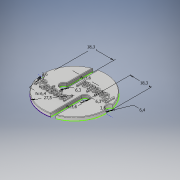
# Autodesk Inventor part: cookie_copied
Saved by Autodesk Inventor 2019 (Build 230136000, 136)
## iProperties
Created: 2019-04-04
Part Number: cookie_copied
Material: Generic
Document SubType Name: Modeling
Designer: jmc
Density: 1 g/cm^3
Appearance: Default
Author: jmc
## iProperties of the stored document cookie_copied_3DPrint.ipt
Created: 2019-04-04
Part Number: cookie_copied_3DPrint
Material: Generic
Document SubType Name: Modeling
Designer: assman
Density: 1 g/cm^3
Appearance: Default
Author: assman
Autodesk Inventor part; units mm, degrees
ref_plane "YZ Plane" through (0, 0, 0) normal (1, 0, 0) x (0, 1, 0)
ref_plane "XZ Plane" through (0, 0, 0) normal (0, 1, 0) x (-1, 0, 0)
ref_plane "XY Plane" through (0, 0, 0) normal (0, 0, 1) x (1, 0, 0)
sketch "Sketch1" plane through (0, 0, 0) normal (0, 1, 0) x (-1, 0, 0)
  line L0 (32.3118, 0) -> (-33.3424, 0) construction
  arc A0 (9.65, -3.1177) -> (6.05, 0) centre (9.2, 0) ccw
  arc A1 (-9.647, 3.1177) -> (-6.047, 0) centre (-9.197, 0) ccw
  line L1 (27.5, 0) -> (27.5, -9.7231) construction
  line L2 (-6.047, 0) -> (-6.047, 26.8269)
  line L3 (-9.647, 3.1177) -> (-9.647, 25.7524)
  arc A2 (-26.6628, -6.734) -> (-27.497, -0.4055) centre (-27.3093, -3.6) ccw
  arc A3 (26.6628, 6.7338) -> (27.497, 0.4054) centre (27.3103, 3.6) ccw
  arc A4 (-9.647, 25.7524) -> (-27.497, -0.4055) centre (0, 0) ccw
  arc A5 (-26.6628, -6.734) -> (6.05, -26.8262) centre (0, 0) ccw
  arc A6 (9.65, -25.7513) -> (27.497, 0.4054) centre (0, 0) ccw
  arc A7 (26.6628, 6.7338) -> (-6.047, 26.8269) centre (0, 0) ccw
  line L4 (-27.497, -0.4055) -> (-27.497, 9.5971) construction
  line L5 (6.05, 0) -> (6.05, -26.8262)
  line L6 (9.65, -25.7513) -> (9.65, -3.1177)
  point P0 (12.35, 0)
  dimension "d1" = 6.3
  dimension "d2" = 6.3
  dimension "d3" = 18.3
  dimension "d6" = 3.6
  dimension "d7" = 6.4
  dimension "d8" = 6.4
  dimension "d11" = 27.5
  dimension "d12" = 18.3
  dimension "d13" = 3.6
  dimension "d14" = 3.6
  dimension "d15" = 3.6
  constraints: 18 point on circle, 14 end point, 8 centre point, 6 point on line, 3 tangent, 3 vertical, 2 perpendicular, 1 coincident, 1 horizontal
  measures "d1" diameter of A0
  measures "d2" diameter of A1
  measures "d3" distance from line of L1 A0.centre
  measures "d6" distance between parallel lines of L2 L3
  measures "d7" diameter of A2
  measures "d8" diameter of A3
  measures "d11" radius of A7
  measures "d12" distance from line of L4 A1.centre
  measures "d13" distance from line of L0 A2.centre
  measures "d14" distance from line of A3.centre L0
  measures "d15" distance between parallel lines of L6 L5
extrude "Extrusion1" add sketch "Sketch1" along normal blind 2.8
sketch "Sketch2" plane through (0, 2.8, 0) normal (0, 1, 0) x (1, 0, 0)
  line L0 (-23.6967, -4.3993) -> (3.8634, -4.3993) construction
  line L1 (3.8634, -4.3993) -> (3.8634, -12.2502) construction
  line L2 (3.8634, -12.2502) -> (-23.6967, -12.2502) construction
  line L3 (-23.6967, -12.2502) -> (-23.6967, -4.3993) construction
  line L4 (23.6967, 4.719) -> (-3.8634, 4.719) construction
  line L5 (-3.8634, 4.719) -> (-3.8634, 12.5699) construction
  line L6 (-3.8634, 12.5699) -> (23.6967, 12.5699) construction
  line L7 (23.6967, 12.5699) -> (23.6967, 4.719) construction
  spline S0 degree 2 poles (-23.1038, -11.4801) (-23.1038, -11.6982) (-22.8993, -12.0662) (-22.654, -12.0798) knots 0 0 0 1 2 2 2
  spline S1 degree 2 poles (-22.654, -12.0798) (-22.3609, -12.0866) (-21.8771, -11.8617) (-21.8634, -11.5483) knots 0 0 0 1 2 2 2
  spline S2 degree 2 poles (-21.8634, -11.5483) (-21.8702, -11.4324) (-21.952, -11.2279) (-21.9793, -11.1666) knots 0 0 0 1 2 2 2
  line L8 (-21.9793, -11.1666) -> (-21.9793, -8.7745)
  line L9 (-21.9793, -8.7745) -> (-18.8784, -11.8345)
  spline S3 degree 2 poles (-18.8784, -11.8345) (-18.8035, -11.9912) (-18.5104, -12.1616) (-18.3673, -12.1616) knots 0 0 0 1 2 2 2
  spline S4 degree 2 poles (-18.3673, -12.1616) (-18.1083, -12.1616) (-17.6926, -11.8209) (-17.6858, -11.5005) knots 0 0 0 1 2 2 2
  spline S5 degree 2 poles (-17.6858, -11.5005) (-17.6858, -11.3915) (-17.863, -11.1325) (-18.1765, -10.9894) (-18.3809, -11.0576) knots 0 0 0 1 2 3 3 3
  line L10 (-18.3809, -11.0576) -> (-21.3319, -8.2429)
  spline S6 degree 2 poles (-21.3319, -8.2429) (-20.296, -8.0249) (-19.0011, -7.2207) (-18.4014, -6.253) (-18.4014, -5.7759) knots 0 0 0 1 2 3 3 3
  spline S7 degree 2 poles (-18.4014, -5.7759) (-18.4082, -5.2102) (-19.1238, -4.5833) (-19.7303, -4.5764) knots 0 0 0 1 2 2 2
  spline S8 degree 2 poles (-19.7303, -4.5764) (-20.3096, -4.5764) (-21.4204, -4.8695) (-21.9793, -5.1557) knots 0 0 0 1 2 2 2
  line L11 (-21.9793, -5.1557) -> (-21.9793, -5.0399)
  spline S9 degree 2 poles (-21.9793, -5.0399) (-21.9043, -4.7741) (-22.1974, -4.4674) (-22.4086, -4.4606) knots 0 0 0 1 2 2 2
  spline S10 degree 2 poles (-22.4086, -4.4606) (-22.654, -4.4674) (-23.0152, -4.74) (-23.022, -4.9581) knots 0 0 0 1 2 2 2
  spline S11 degree 2 poles (-23.022, -4.9581) (-23.022, -5.0467) (-22.9811, -5.2171) (-22.9538, -5.2852) knots 0 0 0 1 2 2 2
  line L12 (-22.9538, -5.2852) -> (-22.9538, -5.4897)
  spline S12 degree 2 poles (-22.9538, -5.4897) (-23.097, -5.5306) (-23.2741, -5.81) (-23.2741, -6.0962) knots 0 0 0 1 2 2 2
  spline S13 degree 2 poles (-23.2741, -6.0962) (-23.2741, -6.3143) (-23.1242, -6.5119) (-23.0424, -6.5119) knots 0 0 0 1 2 2 2
  spline S14 degree 2 poles (-23.0424, -6.5119) (-23.022, -6.5119) (-22.9811, -6.5051) (-22.9538, -6.4847) knots 0 0 0 1 2 2 2
  line L13 (-22.9538, -6.4847) -> (-22.9538, -11.1189)
  spline S15 degree 2 poles (-22.9538, -11.1189) (-22.9947, -11.1939) (-23.097, -11.4051) (-23.1038, -11.4801) knots 0 0 0 1 2 2 2
  spline S16 degree 2 poles (-21.9793, -5.9872) (-21.4204, -5.6873) (-20.3777, -5.4351) (-19.9757, -5.442) knots 0 0 0 1 2 2 2
  spline S17 degree 2 poles (-19.9757, -5.442) (-19.7371, -5.442) (-19.4373, -5.6737) (-19.4305, -5.8918) knots 0 0 0 1 2 2 2
  spline S18 degree 2 poles (-19.4305, -5.8918) (-19.4373, -6.3211) (-20.1051, -6.9822) (-21.2569, -7.4865) (-21.9793, -7.6909) knots 0 0 0 1 2 3 3 3
  line L14 (-21.9793, -7.6909) -> (-21.9793, -5.9872)
  spline S19 degree 2 poles (-15.1097, -6.9004) (-15.7231, -6.9072) (-16.8135, -7.8613) (-17.495, -9.5174) (-17.5086, -10.5873) knots 0 0 0 1 2 3 3 3
  spline S20 degree 2 poles (-17.5086, -10.5873) (-17.495, -11.4801) (-16.7249, -12.2093) (-16.1524, -12.1957) knots 0 0 0 1 2 2 2
  spline S21 degree 2 poles (-16.1524, -12.1957) (-15.6345, -12.1889) (-14.7962, -11.7731) (-14.1965, -11.1871) (-13.8694, -10.6555) (-13.8694, -10.5328) knots 0 0 0 1 2 3 4 4 4
  spline S22 degree 2 poles (-13.8694, -10.5328) (-13.8625, -10.3761) (-14.0466, -10.083) (-14.3464, -10.0694) knots 0 0 0 1 2 2 2
  spline S23 degree 2 poles (-14.3464, -10.0694) (-14.5986, -10.0762) (-14.878, -10.342) (-14.8575, -10.5533) knots 0 0 0 1 2 2 2
  spline S24 degree 2 poles (-14.8575, -10.5533) (-14.9053, -10.7236) (-15.2528, -11.078) (-15.7435, -11.3234) (-16.0161, -11.3302) knots 0 0 0 1 2 3 3 3
  spline S25 degree 2 poles (-16.0161, -11.3302) (-16.2887, -11.337) (-16.5681, -10.9485) (-16.5681, -10.5124) knots 0 0 0 1 2 2 2
  spline S26 degree 2 poles (-16.5681, -10.5124) (-16.5681, -10.3215) (-16.5341, -9.9672) (-16.4863, -9.8036) knots 0 0 0 1 2 2 2
  line L15 (-16.4863, -9.8036) -> (-16.0911, -9.7082)
  spline S27 degree 2 poles (-16.0911, -9.7082) (-15.1301, -9.4901) (-14.1352, -9.0539) (-13.7876, -8.5769) (-13.8012, -8.2975) knots 0 0 0 1 2 3 3 3
  spline S28 degree 2 poles (-13.8012, -8.2975) (-13.8012, -8.0385) (-14.0534, -7.3911) (-14.6327, -6.914) (-15.1097, -6.9004) knots 0 0 0 1 2 3 3 3
  spline S29 degree 2 poles (-15.1642, -7.7795) (-14.9053, -7.7863) (-14.6463, -8.1407) (-14.6463, -8.3792) knots 0 0 0 1 2 2 2
  spline S30 degree 2 poles (-14.6463, -8.3792) (-14.6327, -8.4678) (-14.8712, -8.6382) (-15.5936, -8.8631) (-16.3228, -9.0199) knots 0 0 0 1 2 3 3 3
  spline S31 degree 2 poles (-16.3228, -9.0199) (-16.2342, -8.6996) (-15.9003, -8.1407) (-15.4436, -7.7863) (-15.1642, -7.7795) knots 0 0 0 1 2 3 3 3
  spline S32 degree 2 poles (-11.8317, -7.4933) (-11.8385, -7.3161) (-12.152, -6.9753) (-12.3496, -6.9617) knots 0 0 0 1 2 2 2
  spline S33 degree 2 poles (-12.3496, -6.9617) (-12.6631, -6.9685) (-12.9493, -7.1594) (-13.0175, -7.4592) (-13.0107, -7.6228) knots 0 0 0 1 2 3 3 3
  spline S34 degree 2 poles (-13.0107, -7.6228) (-13.0107, -7.7046) (-12.963, -7.8681) (-12.9084, -7.9226) knots 0 0 0 1 2 2 2
  line L16 (-12.9084, -7.9226) -> (-12.9084, -11.2007)
  spline S35 degree 2 poles (-12.9084, -11.2007) (-12.9493, -11.2348) (-13.0311, -11.4051) (-13.0379, -11.5483) knots 0 0 0 1 2 2 2
  spline S36 degree 2 poles (-13.0379, -11.5483) (-13.0311, -11.78) (-12.779, -12.073) (-12.5609, -12.0798) knots 0 0 0 1 2 2 2
  spline S37 degree 2 poles (-12.5609, -12.0798) (-12.3019, -12.0798) (-11.8385, -11.7936) (-11.818, -11.521) knots 0 0 0 1 2 2 2
  spline S38 degree 2 poles (-11.818, -11.521) (-11.8248, -11.4324) (-11.9066, -11.2688) (-11.9475, -11.2484) knots 0 0 0 1 2 2 2
  line L17 (-11.9475, -11.2484) -> (-11.9475, -7.8749)
  spline S39 degree 2 poles (-11.9475, -7.8749) (-11.9203, -7.834) (-11.8385, -7.6569) (-11.8317, -7.4933) knots 0 0 0 1 2 2 2
  spline S40 degree 2 poles (-12.2337, -4.7741) (-12.5677, -4.7877) (-12.9084, -5.3602) (-12.9084, -5.7827) knots 0 0 0 1 2 2 2
  spline S41 degree 2 poles (-12.9084, -5.7827) (-12.9084, -6.0417) (-12.704, -6.3484) (-12.445, -6.3484) knots 0 0 0 1 2 2 2
  spline S42 degree 2 poles (-12.445, -6.3484) (-12.1792, -6.3415) (-11.7976, -5.7827) (-11.784, -5.292) knots 0 0 0 1 2 2 2
  spline S43 degree 2 poles (-11.784, -5.292) (-11.7908, -5.0399) (-12.0361, -4.7741) (-12.2337, -4.7741) knots 0 0 0 1 2 2 2
  spline S44 degree 2 poles (-8.6695, -6.8936) (-8.9693, -6.9004) (-9.5827, -7.2002) (-10.1006, -7.6364) (-10.2506, -7.8409) knots 0 0 0 1 2 3 3 3
  spline S45 degree 2 poles (-10.2506, -7.8409) (-10.5027, -8.2089) (-10.8503, -8.904) (-11.0343, -9.7832) (-11.0343, -10.417) knots 0 0 0 1 2 3 3 3
  spline S46 degree 2 poles (-11.0343, -10.417) (-11.0343, -11.2211) (-10.2846, -12.2298) (-9.5554, -12.2434) knots 0 0 0 1 2 2 2
  spline S47 degree 2 poles (-9.5554, -12.2434) (-9.1602, -12.2434) (-8.4037, -11.9435) (-8.0902, -11.63) knots 0 0 0 1 2 2 2
  spline S48 degree 2 poles (-8.0902, -11.63) (-7.8449, -11.3642) (-7.5041, -10.8054) (-7.3269, -10.3829) (-7.3269, -10.3215) knots 0 0 0 1 2 3 3 3
  spline S49 degree 2 poles (-7.3269, -10.3215) (-7.3269, -10.1784) (-7.5382, -9.8717) (-7.8176, -9.8581) knots 0 0 0 1 2 2 2
  spline S50 degree 2 poles (-7.8176, -9.8581) (-8.0697, -9.8649) (-8.2469, -10.1716) (-8.2674, -10.4033) knots 0 0 0 1 2 2 2
  spline S51 degree 2 poles (-8.2674, -10.4033) (-8.3628, -10.6418) (-8.6627, -11.0167) (-8.799, -11.1325) knots 0 0 0 1 2 2 2
  spline S52 degree 2 poles (-8.799, -11.1325) (-8.9216, -11.2484) (-9.201, -11.3779) (-9.3646, -11.3779) knots 0 0 0 1 2 2 2
  spline S53 degree 2 poles (-9.3646, -11.3779) (-9.7258, -11.3779) (-10.0734, -10.8327) (-10.0734, -10.2398) knots 0 0 0 1 2 2 2
  spline S54 degree 2 poles (-10.0734, -10.2398) (-10.0734, -9.6741) (-9.8212, -8.7677) (-9.5759, -8.4338) knots 0 0 0 1 2 2 2
  spline S55 degree 2 poles (-9.5759, -8.4338) (-9.351, -8.1066) (-8.8944, -7.7386) (-8.6627, -7.7386) knots 0 0 0 1 2 2 2
  spline S56 degree 2 poles (-8.6627, -7.7386) (-8.4923, -7.7454) (-8.3424, -7.9158) (-8.3151, -8.0181) knots 0 0 0 1 2 2 2
  spline S57 degree 2 poles (-8.3151, -8.0181) (-8.281, -8.1203) (-8.1447, -8.2907) (-7.9743, -8.2975) knots 0 0 0 1 2 2 2
  spline S58 degree 2 poles (-7.9743, -8.2975) (-7.6472, -8.2975) (-7.361, -7.9976) (-7.361, -7.7318) knots 0 0 0 1 2 2 2
  spline S59 degree 2 poles (-7.361, -7.7318) (-7.3814, -7.3911) (-8.1243, -6.9072) (-8.6695, -6.8936) knots 0 0 0 1 2 2 2
  spline S60 degree 2 poles (-4.1784, -11.3302) (-4.2397, -11.3983) (-4.2806, -11.6096) (-4.2806, -11.7118) knots 0 0 0 1 2 2 2
  spline S61 degree 2 poles (-4.2806, -11.7118) (-4.2806, -11.8754) (-3.9875, -12.0798) (-3.7149, -12.0798) knots 0 0 0 1 2 2 2
  spline S62 degree 2 poles (-3.7149, -12.0798) (-3.5105, -12.073) (-3.1356, -11.814) (-3.122, -11.6028) knots 0 0 0 1 2 2 2
  spline S63 degree 2 poles (-3.122, -11.6028) (-3.1288, -11.5278) (-3.2038, -11.4051) (-3.2174, -11.3642) knots 0 0 0 1 2 2 2
  line L18 (-3.2174, -11.3642) -> (-3.2174, -8.0112)
  spline S64 degree 2 poles (-3.2174, -8.0112) (-3.2106, -7.4865) (-3.49, -6.9958) (-3.8444, -6.9958) knots 0 0 0 1 2 2 2
  spline S65 degree 2 poles (-3.8444, -6.9958) (-4.1647, -6.9958) (-4.9416, -7.4728) (-5.4051, -7.9567) knots 0 0 0 1 2 2 2
  line L19 (-5.4051, -7.9567) -> (-5.4255, -7.9567)
  line L20 (-5.4255, -7.9567) -> (-5.4255, -5.2511)
  spline S66 degree 2 poles (-5.4255, -5.2511) (-5.3914, -5.1762) (-5.3437, -5.0126) (-5.3437, -4.9172) knots 0 0 0 1 2 2 2
  spline S67 degree 2 poles (-5.3437, -4.9172) (-5.3574, -4.7196) (-5.6913, -4.4129) (-5.8412, -4.4061) knots 0 0 0 1 2 2 2
  spline S68 degree 2 poles (-5.8412, -4.4061) (-6.107, -4.4061) (-6.4682, -4.6991) (-6.4818, -4.9513) knots 0 0 0 1 2 2 2
  spline S69 degree 2 poles (-6.4818, -4.9513) (-6.475, -5.0399) (-6.3932, -5.2102) (-6.3864, -5.292) knots 0 0 0 1 2 2 2
  line L21 (-6.3864, -5.292) -> (-6.3864, -11.3506)
  spline S70 degree 2 poles (-6.3864, -11.3506) (-6.4273, -11.3983) (-6.4682, -11.5891) (-6.4682, -11.7118) knots 0 0 0 1 2 2 2
  spline S71 degree 2 poles (-6.4682, -11.7118) (-6.475, -11.9094) (-6.2978, -12.0798) (-6.0525, -12.0798) knots 0 0 0 1 2 2 2
  spline S72 degree 2 poles (-6.0525, -12.0798) (-5.7799, -12.0798) (-5.3437, -11.8413) (-5.3301, -11.63) knots 0 0 0 1 2 2 2
  spline S73 degree 2 poles (-5.3301, -11.63) (-5.3369, -11.5278) (-5.3914, -11.3711) (-5.4255, -11.3029) knots 0 0 0 1 2 2 2
  line L22 (-5.4255, -11.3029) -> (-5.4255, -9.0335)
  spline S74 degree 2 poles (-5.4255, -9.0335) (-5.037, -8.4747) (-4.4987, -8.1203) (-4.3487, -8.1339) knots 0 0 0 1 2 2 2
  spline S75 degree 2 poles (-4.3487, -8.1339) (-4.2465, -8.1271) (-4.1784, -8.3384) (-4.1784, -8.5973) knots 0 0 0 1 2 2 2
  line L23 (-4.1784, -8.5973) -> (-4.1784, -11.3302)
  spline S76 degree 2 poles (0.0879, -6.9004) (-0.5255, -6.9072) (-1.6159, -7.8613) (-2.2974, -9.5174) (-2.311, -10.5873) knots 0 0 0 1 2 3 3 3
  spline S77 degree 2 poles (-2.311, -10.5873) (-2.2974, -11.4801) (-1.5273, -12.2093) (-0.9548, -12.1957) knots 0 0 0 1 2 2 2
  spline S78 degree 2 poles (-0.9548, -12.1957) (-0.4369, -12.1889) (0.4014, -11.7731) (1.0011, -11.1871) (1.3282, -10.6555) (1.3282, -10.5328) knots 0 0 0 1 2 3 4 4 4
  spline S79 degree 2 poles (1.3282, -10.5328) (1.335, -10.3761) (1.151, -10.083) (0.8512, -10.0694) knots 0 0 0 1 2 2 2
  spline S80 degree 2 poles (0.8512, -10.0694) (0.599, -10.0762) (0.3196, -10.342) (0.34, -10.5533) knots 0 0 0 1 2 2 2
  spline S81 degree 2 poles (0.34, -10.5533) (0.2923, -10.7236) (-0.0552, -11.078) (-0.5459, -11.3234) (-0.8185, -11.3302) knots 0 0 0 1 2 3 3 3
  spline S82 degree 2 poles (-0.8185, -11.3302) (-1.0911, -11.337) (-1.3705, -10.9485) (-1.3705, -10.5124) knots 0 0 0 1 2 2 2
  spline S83 degree 2 poles (-1.3705, -10.5124) (-1.3705, -10.3215) (-1.3365, -9.9672) (-1.2888, -9.8036) knots 0 0 0 1 2 2 2
  line L24 (-1.2888, -9.8036) -> (-0.8935, -9.7082)
  spline S84 degree 2 poles (-0.8935, -9.7082) (0.0674, -9.4901) (1.0624, -9.0539) (1.41, -8.5769) (1.3964, -8.2975) knots 0 0 0 1 2 3 3 3
  spline S85 degree 2 poles (1.3964, -8.2975) (1.3964, -8.0385) (1.1442, -7.3911) (0.5649, -6.914) (0.0879, -6.9004) knots 0 0 0 1 2 3 3 3
  spline S86 degree 2 poles (0.0334, -7.7795) (0.2923, -7.7863) (0.5513, -8.1407) (0.5513, -8.3792) knots 0 0 0 1 2 2 2
  spline S87 degree 2 poles (0.5513, -8.3792) (0.5649, -8.4678) (0.3264, -8.6382) (-0.396, -8.8631) (-1.1252, -9.0199) knots 0 0 0 1 2 3 3 3
  spline S88 degree 2 poles (-1.1252, -9.0199) (-1.0366, -8.6996) (-0.7027, -8.1407) (-0.2461, -7.7863) (0.0334, -7.7795) knots 0 0 0 1 2 3 3 3
  spline S89 degree 2 poles (2.2891, -11.2484) (2.2551, -11.3234) (2.2005, -11.4733) (2.1937, -11.5551) knots 0 0 0 1 2 2 2
  spline S90 degree 2 poles (2.1937, -11.5551) (2.2005, -11.7936) (2.5345, -12.073) (2.773, -12.0798) knots 0 0 0 1 2 2 2
  spline S91 degree 2 poles (2.773, -12.0798) (3.0456, -12.0662) (3.4068, -11.7731) (3.4136, -11.6164) knots 0 0 0 1 2 2 2
  spline S92 degree 2 poles (3.4136, -11.6164) (3.4136, -11.5278) (3.325, -11.3642) (3.2501, -11.3029) knots 0 0 0 1 2 2 2
  line L25 (3.2501, -11.3029) -> (3.2501, -5.4556)
  spline S93 degree 2 poles (3.2501, -5.4556) (3.3318, -5.3465) (3.4204, -5.0876) (3.4204, -4.9513) knots 0 0 0 1 2 2 2
  spline S94 degree 2 poles (3.4204, -4.9513) (3.4136, -4.6855) (3.032, -4.4265) (2.8071, -4.4265) knots 0 0 0 1 2 2 2
  spline S95 degree 2 poles (2.8071, -4.4265) (2.4323, -4.4197) (2.1733, -4.6582) (2.1869, -4.9922) knots 0 0 0 1 2 2 2
  spline S96 degree 2 poles (2.1869, -4.9922) (2.1869, -5.1012) (2.2551, -5.3057) (2.2891, -5.3874) knots 0 0 0 1 2 2 2
  line L26 (2.2891, -5.3874) -> (2.2891, -11.2484)
  spline S97 degree 2 poles (23.1038, 11.7998) (23.1038, 12.0179) (22.8993, 12.3859) (22.654, 12.3996) knots 0 0 0 1 2 2 2
  spline S98 degree 2 poles (22.654, 12.3996) (22.3609, 12.4064) (21.8771, 12.1815) (21.8634, 11.868) knots 0 0 0 1 2 2 2
  spline S99 degree 2 poles (21.8634, 11.868) (21.8702, 11.7521) (21.952, 11.5477) (21.9793, 11.4864) knots 0 0 0 1 2 2 2
  line L27 (21.9793, 11.4864) -> (21.9793, 9.0943)
  line L28 (21.9793, 9.0943) -> (18.8784, 12.1542)
  spline S100 degree 2 poles (18.8784, 12.1542) (18.8035, 12.311) (18.5104, 12.4814) (18.3673, 12.4814) knots 0 0 0 1 2 2 2
  spline S101 degree 2 poles (18.3673, 12.4814) (18.1083, 12.4814) (17.6926, 12.1406) (17.6858, 11.8203) knots 0 0 0 1 2 2 2
  spline S102 degree 2 poles (17.6858, 11.8203) (17.6858, 11.7112) (17.863, 11.4523) (18.1765, 11.3092) (18.3809, 11.3773) knots 0 0 0 1 2 3 3 3
  line L29 (18.3809, 11.3773) -> (21.3319, 8.5627)
  spline S103 degree 2 poles (21.3319, 8.5627) (20.296, 8.3446) (19.0011, 7.5404) (18.4014, 6.5727) (18.4014, 6.0956) knots 0 0 0 1 2 3 3 3
  spline S104 degree 2 poles (18.4014, 6.0956) (18.4082, 5.53) (19.1238, 4.903) (19.7303, 4.8962) knots 0 0 0 1 2 2 2
  spline S105 degree 2 poles (19.7303, 4.8962) (20.3096, 4.8962) (21.4204, 5.1892) (21.9793, 5.4755) knots 0 0 0 1 2 2 2
  line L30 (21.9793, 5.4755) -> (21.9793, 5.3596)
  spline S106 degree 2 poles (21.9793, 5.3596) (21.9043, 5.0938) (22.1974, 4.7871) (22.4086, 4.7803) knots 0 0 0 1 2 2 2
  spline S107 degree 2 poles (22.4086, 4.7803) (22.654, 4.7871) (23.0152, 5.0598) (23.022, 5.2778) knots 0 0 0 1 2 2 2
  spline S108 degree 2 poles (23.022, 5.2778) (23.022, 5.3664) (22.9811, 5.5368) (22.9538, 5.605) knots 0 0 0 1 2 2 2
  line L31 (22.9538, 5.605) -> (22.9538, 5.8094)
  spline S109 degree 2 poles (22.9538, 5.8094) (23.097, 5.8503) (23.2741, 6.1297) (23.2741, 6.4159) knots 0 0 0 1 2 2 2
  spline S110 degree 2 poles (23.2741, 6.4159) (23.2741, 6.634) (23.1242, 6.8317) (23.0424, 6.8317) knots 0 0 0 1 2 2 2
  spline S111 degree 2 poles (23.0424, 6.8317) (23.022, 6.8317) (22.9811, 6.8249) (22.9538, 6.8044) knots 0 0 0 1 2 2 2
  line L32 (22.9538, 6.8044) -> (22.9538, 11.4386)
  spline S112 degree 2 poles (22.9538, 11.4386) (22.9947, 11.5136) (23.097, 11.7249) (23.1038, 11.7998) knots 0 0 0 1 2 2 2
  spline S113 degree 2 poles (21.9793, 6.3069) (21.4204, 6.007) (20.3777, 5.7549) (19.9757, 5.7617) knots 0 0 0 1 2 2 2
  spline S114 degree 2 poles (19.9757, 5.7617) (19.7371, 5.7617) (19.4373, 5.9934) (19.4305, 6.2115) knots 0 0 0 1 2 2 2
  spline S115 degree 2 poles (19.4305, 6.2115) (19.4373, 6.6408) (20.1051, 7.3019) (21.2569, 7.8062) (21.9793, 8.0107) knots 0 0 0 1 2 3 3 3
  line L33 (21.9793, 8.0107) -> (21.9793, 6.3069)
  spline S116 degree 2 poles (15.1097, 7.2201) (15.7231, 7.2269) (16.8135, 8.181) (17.495, 9.8371) (17.5086, 10.9071) knots 0 0 0 1 2 3 3 3
  spline S117 degree 2 poles (17.5086, 10.9071) (17.495, 11.7998) (16.7249, 12.5291) (16.1524, 12.5154) knots 0 0 0 1 2 2 2
  spline S118 degree 2 poles (16.1524, 12.5154) (15.6345, 12.5086) (14.7962, 12.0929) (14.1965, 11.5068) (13.8694, 10.9752) (13.8694, 10.8526) knots 0 0 0 1 2 3 4 4 4
  spline S119 degree 2 poles (13.8694, 10.8526) (13.8625, 10.6958) (14.0466, 10.4028) (14.3464, 10.3891) knots 0 0 0 1 2 2 2
  spline S120 degree 2 poles (14.3464, 10.3891) (14.5986, 10.3959) (14.878, 10.6617) (14.8575, 10.873) knots 0 0 0 1 2 2 2
  spline S121 degree 2 poles (14.8575, 10.873) (14.9053, 11.0434) (15.2528, 11.3978) (15.7435, 11.6431) (16.0161, 11.6499) knots 0 0 0 1 2 3 3 3
  spline S122 degree 2 poles (16.0161, 11.6499) (16.2887, 11.6567) (16.5681, 11.2683) (16.5681, 10.8321) knots 0 0 0 1 2 2 2
  spline S123 degree 2 poles (16.5681, 10.8321) (16.5681, 10.6413) (16.5341, 10.2869) (16.4863, 10.1233) knots 0 0 0 1 2 2 2
  line L34 (16.4863, 10.1233) -> (16.0911, 10.0279)
  spline S124 degree 2 poles (16.0911, 10.0279) (15.1301, 9.8098) (14.1352, 9.3737) (13.7876, 8.8966) (13.8012, 8.6172) knots 0 0 0 1 2 3 3 3
  spline S125 degree 2 poles (13.8012, 8.6172) (13.8012, 8.3582) (14.0534, 7.7108) (14.6327, 7.2338) (15.1097, 7.2201) knots 0 0 0 1 2 3 3 3
  spline S126 degree 2 poles (15.1642, 8.0993) (14.9053, 8.1061) (14.6463, 8.4605) (14.6463, 8.699) knots 0 0 0 1 2 2 2
  spline S127 degree 2 poles (14.6463, 8.699) (14.6327, 8.7876) (14.8712, 8.958) (15.5936, 9.1829) (16.3228, 9.3396) knots 0 0 0 1 2 3 3 3
  spline S128 degree 2 poles (16.3228, 9.3396) (16.2342, 9.0193) (15.9003, 8.4605) (15.4436, 8.1061) (15.1642, 8.0993) knots 0 0 0 1 2 3 3 3
  spline S129 degree 2 poles (11.8317, 7.813) (11.8385, 7.6358) (12.152, 7.2951) (12.3496, 7.2815) knots 0 0 0 1 2 2 2
  spline S130 degree 2 poles (12.3496, 7.2815) (12.6631, 7.2883) (12.9493, 7.4791) (13.0175, 7.779) (13.0107, 7.9425) knots 0 0 0 1 2 3 3 3
  spline S131 degree 2 poles (13.0107, 7.9425) (13.0107, 8.0243) (12.963, 8.1879) (12.9084, 8.2424) knots 0 0 0 1 2 2 2
  line L35 (12.9084, 8.2424) -> (12.9084, 11.5204)
  spline S132 degree 2 poles (12.9084, 11.5204) (12.9493, 11.5545) (13.0311, 11.7249) (13.0379, 11.868) knots 0 0 0 1 2 2 2
  spline S133 degree 2 poles (13.0379, 11.868) (13.0311, 12.0997) (12.779, 12.3928) (12.5609, 12.3996) knots 0 0 0 1 2 2 2
  spline S134 degree 2 poles (12.5609, 12.3996) (12.3019, 12.3996) (11.8385, 12.1133) (11.818, 11.8407) knots 0 0 0 1 2 2 2
  spline S135 degree 2 poles (11.818, 11.8407) (11.8248, 11.7521) (11.9066, 11.5886) (11.9475, 11.5681) knots 0 0 0 1 2 2 2
  line L36 (11.9475, 11.5681) -> (11.9475, 8.1947)
  spline S136 degree 2 poles (11.9475, 8.1947) (11.9203, 8.1538) (11.8385, 7.9766) (11.8317, 7.813) knots 0 0 0 1 2 2 2
  spline S137 degree 2 poles (12.2337, 5.0938) (12.5677, 5.1075) (12.9084, 5.6799) (12.9084, 6.1025) knots 0 0 0 1 2 2 2
  spline S138 degree 2 poles (12.9084, 6.1025) (12.9084, 6.3614) (12.704, 6.6681) (12.445, 6.6681) knots 0 0 0 1 2 2 2
  spline S139 degree 2 poles (12.445, 6.6681) (12.1792, 6.6613) (11.7976, 6.1025) (11.784, 5.6118) knots 0 0 0 1 2 2 2
  spline S140 degree 2 poles (11.784, 5.6118) (11.7908, 5.3596) (12.0361, 5.0938) (12.2337, 5.0938) knots 0 0 0 1 2 2 2
  spline S141 degree 2 poles (8.6695, 7.2133) (8.9693, 7.2201) (9.5827, 7.52) (10.1006, 7.9562) (10.2506, 8.1606) knots 0 0 0 1 2 3 3 3
  spline S142 degree 2 poles (10.2506, 8.1606) (10.5027, 8.5286) (10.8503, 9.2238) (11.0343, 10.1029) (11.0343, 10.7367) knots 0 0 0 1 2 3 3 3
  spline S143 degree 2 poles (11.0343, 10.7367) (11.0343, 11.5409) (10.2846, 12.5495) (9.5554, 12.5631) knots 0 0 0 1 2 2 2
  spline S144 degree 2 poles (9.5554, 12.5631) (9.1602, 12.5631) (8.4037, 12.2633) (8.0902, 11.9498) knots 0 0 0 1 2 2 2
  spline S145 degree 2 poles (8.0902, 11.9498) (7.8449, 11.684) (7.5041, 11.1252) (7.3269, 10.7026) (7.3269, 10.6413) knots 0 0 0 1 2 3 3 3
  spline S146 degree 2 poles (7.3269, 10.6413) (7.3269, 10.4982) (7.5382, 10.1915) (7.8176, 10.1779) knots 0 0 0 1 2 2 2
  spline S147 degree 2 poles (7.8176, 10.1779) (8.0697, 10.1847) (8.2469, 10.4914) (8.2674, 10.7231) knots 0 0 0 1 2 2 2
  spline S148 degree 2 poles (8.2674, 10.7231) (8.3628, 10.9616) (8.6627, 11.3364) (8.799, 11.4523) knots 0 0 0 1 2 2 2
  spline S149 degree 2 poles (8.799, 11.4523) (8.9216, 11.5681) (9.201, 11.6976) (9.3646, 11.6976) knots 0 0 0 1 2 2 2
  spline S150 degree 2 poles (9.3646, 11.6976) (9.7258, 11.6976) (10.0734, 11.1524) (10.0734, 10.5595) knots 0 0 0 1 2 2 2
  spline S151 degree 2 poles (10.0734, 10.5595) (10.0734, 9.9939) (9.8212, 9.0875) (9.5759, 8.7535) knots 0 0 0 1 2 2 2
  spline S152 degree 2 poles (9.5759, 8.7535) (9.351, 8.4264) (8.8944, 8.0584) (8.6627, 8.0584) knots 0 0 0 1 2 2 2
  spline S153 degree 2 poles (8.6627, 8.0584) (8.4923, 8.0652) (8.3424, 8.2356) (8.3151, 8.3378) knots 0 0 0 1 2 2 2
  spline S154 degree 2 poles (8.3151, 8.3378) (8.281, 8.44) (8.1447, 8.6104) (7.9743, 8.6172) knots 0 0 0 1 2 2 2
  spline S155 degree 2 poles (7.9743, 8.6172) (7.6472, 8.6172) (7.361, 8.3174) (7.361, 8.0516) knots 0 0 0 1 2 2 2
  spline S156 degree 2 poles (7.361, 8.0516) (7.3814, 7.7108) (8.1243, 7.2269) (8.6695, 7.2133) knots 0 0 0 1 2 2 2
  spline S157 degree 2 poles (4.1784, 11.6499) (4.2397, 11.7181) (4.2806, 11.9293) (4.2806, 12.0316) knots 0 0 0 1 2 2 2
  spline S158 degree 2 poles (4.2806, 12.0316) (4.2806, 12.1951) (3.9875, 12.3996) (3.7149, 12.3996) knots 0 0 0 1 2 2 2
  spline S159 degree 2 poles (3.7149, 12.3996) (3.5105, 12.3928) (3.1356, 12.1338) (3.122, 11.9225) knots 0 0 0 1 2 2 2
  spline S160 degree 2 poles (3.122, 11.9225) (3.1288, 11.8476) (3.2038, 11.7249) (3.2174, 11.684) knots 0 0 0 1 2 2 2
  line L37 (3.2174, 11.684) -> (3.2174, 8.331)
  spline S161 degree 2 poles (3.2174, 8.331) (3.2106, 7.8062) (3.49, 7.3155) (3.8444, 7.3155) knots 0 0 0 1 2 2 2
  spline S162 degree 2 poles (3.8444, 7.3155) (4.1647, 7.3155) (4.9416, 7.7926) (5.4051, 8.2765) knots 0 0 0 1 2 2 2
  line L38 (5.4051, 8.2765) -> (5.4255, 8.2765)
  line L39 (5.4255, 8.2765) -> (5.4255, 5.5709)
  spline S163 degree 2 poles (5.4255, 5.5709) (5.3914, 5.4959) (5.3437, 5.3324) (5.3437, 5.2369) knots 0 0 0 1 2 2 2
  spline S164 degree 2 poles (5.3437, 5.2369) (5.3574, 5.0393) (5.6913, 4.7326) (5.8412, 4.7258) knots 0 0 0 1 2 2 2
  spline S165 degree 2 poles (5.8412, 4.7258) (6.107, 4.7258) (6.4682, 5.0189) (6.4818, 5.271) knots 0 0 0 1 2 2 2
  spline S166 degree 2 poles (6.4818, 5.271) (6.475, 5.3596) (6.3932, 5.53) (6.3864, 5.6118) knots 0 0 0 1 2 2 2
  line L40 (6.3864, 5.6118) -> (6.3864, 11.6704)
  spline S167 degree 2 poles (6.3864, 11.6704) (6.4273, 11.7181) (6.4682, 11.9089) (6.4682, 12.0316) knots 0 0 0 1 2 2 2
  spline S168 degree 2 poles (6.4682, 12.0316) (6.475, 12.2292) (6.2978, 12.3996) (6.0525, 12.3996) knots 0 0 0 1 2 2 2
  spline S169 degree 2 poles (6.0525, 12.3996) (5.7799, 12.3996) (5.3437, 12.161) (5.3301, 11.9498) knots 0 0 0 1 2 2 2
  spline S170 degree 2 poles (5.3301, 11.9498) (5.3369, 11.8476) (5.3914, 11.6908) (5.4255, 11.6227) knots 0 0 0 1 2 2 2
  line L41 (5.4255, 11.6227) -> (5.4255, 9.3532)
  spline S171 degree 2 poles (5.4255, 9.3532) (5.037, 8.7944) (4.4987, 8.44) (4.3487, 8.4537) knots 0 0 0 1 2 2 2
  spline S172 degree 2 poles (4.3487, 8.4537) (4.2465, 8.4468) (4.1784, 8.6581) (4.1784, 8.9171) knots 0 0 0 1 2 2 2
  line L42 (4.1784, 8.9171) -> (4.1784, 11.6499)
  spline S173 degree 2 poles (-0.0879, 7.2201) (0.5255, 7.2269) (1.6159, 8.181) (2.2974, 9.8371) (2.311, 10.9071) knots 0 0 0 1 2 3 3 3
  spline S174 degree 2 poles (2.311, 10.9071) (2.2974, 11.7998) (1.5273, 12.5291) (0.9548, 12.5154) knots 0 0 0 1 2 2 2
  spline S175 degree 2 poles (0.9548, 12.5154) (0.4369, 12.5086) (-0.4014, 12.0929) (-1.0011, 11.5068) (-1.3282, 10.9752) (-1.3282, 10.8526) knots 0 0 0 1 2 3 4 4 4
  spline S176 degree 2 poles (-1.3282, 10.8526) (-1.335, 10.6958) (-1.151, 10.4028) (-0.8512, 10.3891) knots 0 0 0 1 2 2 2
  spline S177 degree 2 poles (-0.8512, 10.3891) (-0.599, 10.3959) (-0.3196, 10.6617) (-0.34, 10.873) knots 0 0 0 1 2 2 2
  spline S178 degree 2 poles (-0.34, 10.873) (-0.2923, 11.0434) (0.0552, 11.3978) (0.5459, 11.6431) (0.8185, 11.6499) knots 0 0 0 1 2 3 3 3
  spline S179 degree 2 poles (0.8185, 11.6499) (1.0911, 11.6567) (1.3705, 11.2683) (1.3705, 10.8321) knots 0 0 0 1 2 2 2
  spline S180 degree 2 poles (1.3705, 10.8321) (1.3705, 10.6413) (1.3365, 10.2869) (1.2888, 10.1233) knots 0 0 0 1 2 2 2
  line L43 (1.2888, 10.1233) -> (0.8935, 10.0279)
  spline S181 degree 2 poles (0.8935, 10.0279) (-0.0674, 9.8098) (-1.0624, 9.3737) (-1.41, 8.8966) (-1.3964, 8.6172) knots 0 0 0 1 2 3 3 3
  spline S182 degree 2 poles (-1.3964, 8.6172) (-1.3964, 8.3582) (-1.1442, 7.7108) (-0.5649, 7.2338) (-0.0879, 7.2201) knots 0 0 0 1 2 3 3 3
  spline S183 degree 2 poles (-0.0334, 8.0993) (-0.2923, 8.1061) (-0.5513, 8.4605) (-0.5513, 8.699) knots 0 0 0 1 2 2 2
  spline S184 degree 2 poles (-0.5513, 8.699) (-0.5649, 8.7876) (-0.3264, 8.958) (0.396, 9.1829) (1.1252, 9.3396) knots 0 0 0 1 2 3 3 3
  spline S185 degree 2 poles (1.1252, 9.3396) (1.0366, 9.0193) (0.7027, 8.4605) (0.2461, 8.1061) (-0.0334, 8.0993) knots 0 0 0 1 2 3 3 3
  spline S186 degree 2 poles (-2.2891, 11.5681) (-2.2551, 11.6431) (-2.2005, 11.793) (-2.1937, 11.8748) knots 0 0 0 1 2 2 2
  spline S187 degree 2 poles (-2.1937, 11.8748) (-2.2005, 12.1133) (-2.5345, 12.3928) (-2.773, 12.3996) knots 0 0 0 1 2 2 2
  spline S188 degree 2 poles (-2.773, 12.3996) (-3.0456, 12.3859) (-3.4068, 12.0929) (-3.4136, 11.9361) knots 0 0 0 1 2 2 2
  spline S189 degree 2 poles (-3.4136, 11.9361) (-3.4136, 11.8476) (-3.325, 11.684) (-3.2501, 11.6227) knots 0 0 0 1 2 2 2
  line L44 (-3.2501, 11.6227) -> (-3.2501, 5.7753)
  spline S190 degree 2 poles (-3.2501, 5.7753) (-3.3318, 5.6663) (-3.4204, 5.4073) (-3.4204, 5.271) knots 0 0 0 1 2 2 2
  spline S191 degree 2 poles (-3.4204, 5.271) (-3.4136, 5.0052) (-3.032, 4.7463) (-2.8071, 4.7463) knots 0 0 0 1 2 2 2
  spline S192 degree 2 poles (-2.8071, 4.7463) (-2.4323, 4.7394) (-2.1733, 4.978) (-2.1869, 5.3119) knots 0 0 0 1 2 2 2
  spline S193 degree 2 poles (-2.1869, 5.3119) (-2.1869, 5.421) (-2.2551, 5.6254) (-2.2891, 5.7072) knots 0 0 0 1 2 2 2
  line L45 (-2.2891, 5.7072) -> (-2.2891, 11.5681)
  point P0 (0, 0)
  constraints: 4 other
extrude "Extrusion2" add sketch "Sketch2" along normal blind 1
fillet "Fillet1" radius 0.4 12 edges at (14.3926, 2.8, -23.433) (24.1367, 2.8, -3.1818) (22.7152, 2.8, 15.5007) (9.647, 2.8, 14.435) (6.047, 2.8, 13.4135) (11.2592, 2.8, -2.3812) (-14.394, 2.8, 23.4321) (-24.1378, 2.8, 3.1818) (-22.716, 2.8, -15.4994) (-9.65, 2.8, -14.4345) (-6.05, 2.8, -13.4131) (-11.2622, 2.8, 2.3812)
equation "\"d6\" = d5"
equation "\"d8\" = d7"
equation "\"d15\" = d6"
equation "\"d5\" = 3.6"
body "Solid1"
